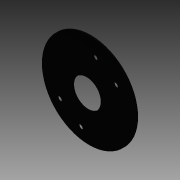
# Autodesk Inventor part: Upper Hub Plate
Saved by Autodesk Inventor 2015 SP1 (Build 190203100, 203)
## iProperties
Created: 2015-01-24
Part Number: Upper Hub Plate
Material: Aluminum
Document SubType Name: Sheet Metal
Designer: Brian
Density: 2.7 g/cm^3
Appearance: Anodized - Black
Sheet Metal Rule: Default
Author: Brian
Autodesk Inventor part; units mm, degrees
ref_plane "YZ Plane" through (0, 0, 0) normal (1, 0, 0) x (0, 1, 0)
ref_plane "XZ Plane" through (0, 0, 0) normal (0, 1, 0) x (-1, 0, 0)
ref_plane "XY Plane" through (0, 0, 0) normal (0, 0, 1) x (1, 0, 0)
sketch "Sketch1" plane through (0, 0, 0) normal (0, 0, 1) x (1, 0, 0)
  circle A0 centre (8.602, 43.9333) radius 18.288 construction
  circle A1 centre (-28.4777, 18.849) radius 3.302 projected
  circle A2 centre (0, 0) radius 3.302 projected
  circle A3 centre (19.9674, 91.247) radius 3.302 projected
  circle A4 centre (47.7138, 72.8821) radius 3.302 projected
  ellipse E0 centre (12.1068, 49.2285) end of major axis (47.4715, 102.6587) minor radius 35.9584 construction
  circle A5 centre (8.602, 43.9333) radius 19.304
  circle A6 centre (8.602, 43.9333) radius 19.05 construction
  line L0 (47.4715, 102.6587) -> (-23.2579, -4.2018) construction
  line L1 (19.9674, 91.247) -> (47.4715, 102.6587) construction
  line L2 (47.7138, 72.8821) -> (47.4715, 102.6587) construction
  circle A7 centre (12.1068, 49.2285) radius 64.0738
  point P0 (0, 0)
  dimension "d3" = 38.1
  dimension "d4" = 0.254
  constraints: 6 end point, 3 centre point, 2 coincident, 2 midpoint, 2 point on circle, 1 equal length, 3 other
  measures "d3" diameter of A6
  measures "d4" radial gap between concentric circles of A6 A5
extrude "Extrusion1" add sketch "Sketch1" along normal blind 2.286
equation "\"BendRadius\" = Thickness"
equation "\"BendReliefWidth\" = Thickness"
equation "\"BendReliefDepth\" = 0.5 * Thickness"
equation "\"CornerReliefSize\" = 4 * Thickness"
equation "\"MinimumRemnant\" = 2 * Thickness"
equation "\"TransitionRadius\" = BendRadius"
equation "\"JacobiRadiusSize\" = BendRadius"
equation "\"GapSize\" = Thickness"
equation "\"Thickness\" = 2.286"
body "Solid1"
